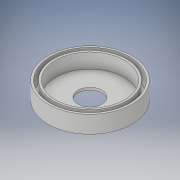
# Autodesk Inventor part: Base
Saved by Autodesk Inventor 2019 (Build 230136000, 136)
## iProperties
Created: 2020-03-27
Part Number: Base
Material: Generic
Document SubType Name: Modeling
Designer: Sergio
Density: 1 g/cm^3
Appearance: Default
Author: Sergio
Autodesk Inventor part; units mm, degrees
ref_plane "YZ Plane" through (0, 0, 0) normal (1, 0, 0) x (0, 1, 0)
ref_plane "XZ Plane" through (0, 0, 0) normal (0, 1, 0) x (-1, 0, 0)
ref_plane "XY Plane" through (0, 0, 0) normal (0, 0, 1) x (1, 0, 0)
sketch "Sketch1" plane through (0, 0, 0) normal (1, 0, 0) x (0, 1, 0)
  line L0 (0, 0) -> (0, 60.75)
  line L1 (0, 60.75) -> (25, 60.75)
  line L2 (25, 60.75) -> (25, 57.75)
  line L3 (25, 57.75) -> (3.5, 57.75)
  line L4 (3.5, 57.75) -> (3.5, 52.75)
  line L5 (3.5, 52.75) -> (25, 52.75)
  line L6 (25, 52.75) -> (25, 49.75)
  line L7 (25, 49.75) -> (3.5, 49.75)
  line L8 (3.5, 49.75) -> (3.5, 0)
  line L9 (3.5, 0) -> (0, 0)
  line L10 (25, 57.75) -> (25, 52.75) construction
  line L11 (3.5, 55.25) -> (25, 55.25) construction
  line L12 (-5, 0) -> (30, 0) projected
  dimension "d1" = 25
  dimension "d2" = 3
  dimension "d4" = 5
  dimension "d7" = 3.5
  dimension "d8" = 55.25
  dimension "d9" = 3.5
  constraints: 24 end point, 6 perpendicular, 4 vertical, 2 midpoint, 2 point on line, 1 collinear
  measures "d1" distance of L0.end L1.end
  measures "d2" distance of L1.end L2.end
  measures "d4" distance of L3.end L4.end
  measures "d7" distance between parallel lines of L0 L8
  measures "d8" distance from line of L0.start L11
  measures "d9" distance between parallel lines of L0 L4
revolve "Revolution1" add sketch "Sketch1" angle 360 about axis through (0, -10, 0) along (0, 1, 0)
sketch "Sketch2" plane through (0, 3.5, 0) normal (0, 1, 0) x (1, 0, 0)
  circle A0 centre (0, 0) radius 17.5
  dimension "d11" = 35
  constraints: 1 centre point, 1 coincident
  measures "d11" diameter of A0
extrude "Extrusion1" cut sketch "Sketch2" against normal blind 40
body "Solid1"
